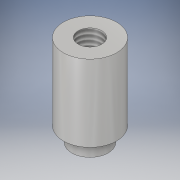
# Autodesk Inventor part: Keystone24884
Saved by Autodesk Inventor 2019 (Build 230136000, 136)
## iProperties
Created: 2019-04-28
Part Number: Keystone24884
Material: Aluminum 6061
Document SubType Name: Modeling
Designer: Lars Larsen
Density: 2.7 g/cm^3
Appearance: Aluminum - Polished
Author: Lars Larsen
Autodesk Inventor part; units mm, degrees
ref_plane "YZ Plane" through (0, 0, 0) normal (1, 0, 0) x (0, 1, 0)
ref_plane "XZ Plane" through (0, 0, 0) normal (0, 1, 0) x (-1, 0, 0)
ref_plane "XY Plane" through (0, 0, 0) normal (0, 0, 1) x (1, 0, 0)
sketch "Sketch1" plane through (0, 0, 0) normal (0, 1, 0) x (-1, 0, 0)
  circle A0 centre (0, 0) radius 2.78
  circle A1 centre (0, 0) radius 2.045
  dimension "d0" = 5.56
  dimension "d1" = 4.09
  constraints: 2 centre point, 2 coincident
  measures "d0" diameter of A0
  measures "d1" diameter of A1
extrude "Extrusion1" add sketch "Sketch1" along normal blind 8
sketch "Sketch2" plane through (0, 0, 0) normal (0, -1, 0) x (1, 0, 0)
  circle A0 centre (0, 0) radius 1.905
  dimension "d4" = 3.81
  constraints: 1 centre point, 1 coincident
  measures "d4" diameter of A0
extrude "Extrusion2" add sketch "Sketch2" along normal blind 1.524
sketch "Sketch3" plane through (0, 0, 0) normal (0, -1, 0) x (1, 0, 0)
  circle A0 centre (0, 0) radius 2.78
  constraints: 1 centre point, 1 coincident
extrude "Extrusion3" add sketch "Sketch3" against normal up to surface (8 mm away)
sketch "Sketch4" plane through (0, 8, 0) normal (0, 1, 0) x (1, 0, 0)
  point P0 (0, 0)
  point P1 (0, 0)
  constraints: 1 coincident
hole "Hole1" at (0, 8, 0) direction (0, -1, 0) diameter 2.4638 end through all
body "Solid1"
